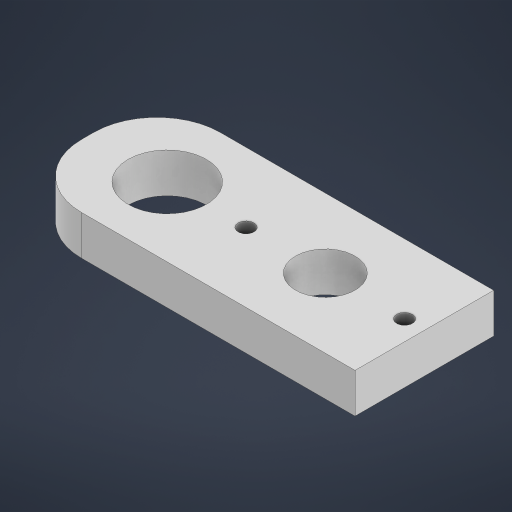
# Autodesk Inventor part: Bear_fix
Saved by Autodesk Inventor 2023 (Build 270158000, 158)
## iProperties
Created: 2023-11-05
Part Number: Bear_fix
Material: Generic
Document SubType Name: Modeling
Designer: Abhinav
Density: 1 g/cm^3
Appearance: Default
Author: Abhinav
Autodesk Inventor part; units mm, degrees
ref_plane "YZ Plane" through (0, 0, 0) normal (1, 0, 0) x (0, 1, 0)
ref_plane "XZ Plane" through (0, 0, 0) normal (0, 1, 0) x (-1, 0, 0)
ref_plane "XY Plane" through (0, 0, 0) normal (0, 0, 1) x (1, 0, 0)
sketch "Sketch1" plane through (0, 0, 0) normal (0, 1, 0) x (-1, 0, 0)
  circle A0 centre (0, 0) radius 4
  circle A1 centre (-20, 0) radius 2
  circle A2 centre (20, 0) radius 2
  circle A3 centre (0, 0) radius 7.5
  line L0 (0, 0) -> (20, 0) construction
  circle A4 centre (0, 0) radius 3.9303 construction
  line L1 (0, 0) -> (39.9, 0) construction
  circle A5 centre (39.9, 0) radius 9.875
  line L2 (-20, 0) -> (-25, 0)
  line L3 (-25, 0) -> (-25, 17.5)
  line L4 (-25, 17.5) -> (60, 17.5)
  line L5 (60, 17.5) -> (60, -17.5)
  line L6 (60, -17.5) -> (-25, -17.5)
  line L7 (-25, -17.5) -> (-25, 17.5)
  dimension "d0" = 8
  dimension "d1" = 39.9
  dimension "d2" = 19.75
  dimension "d3" = 5
  dimension "d4" = 17.5
  dimension "d5" = 85
  dimension "d6" = 35
  constraints: 16 end point, 6 centre point, 3 coincident, 3 horizontal, 2 parallel, 2 perpendicular, 1 equal radius, 1 other
  measures "d0" diameter of A0
  measures "d1" distance of L0.start L1.end
  measures "d2" diameter of A5
  measures "d3" distance of L2.start L2.end
  measures "d4" distance of L2.end L3.end
  measures "d5" distance of L5.end L6.end
  measures "d6" distance of L4.end L5.end
extrude "Extrusion1" add sketch "Sketch1" along normal blind 10 contours L3 L4 L5 L6 L7
fillet "Fillet1" radius 16 2 edges at (-60, 5, -17.5) (-60, 5, 17.5)
body "Solid1"
